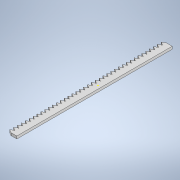
# Autodesk Inventor part: modelGateZoubkouváTyč
Saved by Autodesk Inventor 2020 (Build 240168000, 168)
## iProperties
Created: 2023-11-04
Part Number: modelGateZoubkouváTyč
Material: Generic
Document SubType Name: Sheet Metal
Designer: jirka
Density: 1 g/cm^3
Sheet Metal Rule: Default_mm
Appearance: Default
Author: jirka
Autodesk Inventor part; units mm, degrees
ref_plane "YZ Plane" through (0, 0, 0) normal (1, 0, 0) x (0, 1, 0)
ref_plane "XZ Plane" through (0, 0, 0) normal (0, 1, 0) x (-1, 0, 0)
ref_plane "XY Plane" through (0, 0, 0) normal (0, 0, 1) x (1, 0, 0)
sketch "Sketch1" plane through (0, 0, 0) normal (0, 1, 0) x (-1, 0, 0)
  line L0 (2.25, 55) -> (-2.25, 55)
  line L1 (-2.25, 55) -> (-2.25, -55)
  line L2 (-2.25, -55) -> (2.25, -55)
  line L3 (2.25, -55) -> (2.25, 55)
  point P0 (0, 0)
  dimension "d0" = 4.5
  dimension "d1" = 110
  dimension "d2" = 2.25
  dimension "d3" = 55
  constraints: 8 end point, 2 parallel, 1 horizontal, 1 perpendicular
  measures "d0" distance of L2.end L1.end
  measures "d1" distance of L1.end L0.end
  measures "d2" distance from line of L3 point (0, 0)
  measures "d3" distance from line of L0 point (0, 0)
extrude "Extrusion1" add sketch "Sketch1" along normal blind 2
sketch "Sketch2" plane through (0, 2, 0) normal (0, 1, 0) x (1, 0, 0)
  line L0 (-2.25, 55) -> (-2.25, -55) projected
  line L1 (-2.25, -55) -> (-3.2, -55)
  line L2 (-3.2, -55) -> (-3.2, -53)
  line L3 (-3.2, -53) -> (-2.25, -53)
  line L4 (-2.25, -53) -> (-2.25, -55)
  line L5 (-2.25, -55) -> (-3.2, -54)
  line L6 (-2.25, -53) -> (-3.2, -54)
  line L7 (-3.2, -54) -> (-2.25, -54)
  line L8 (-2.25, -54) -> (-2.513, -54)
  circle A0 centre (-2.513, -54) radius 0.5
  point P0 (0, 0)
  point P1 (-2.9043, -53.6887)
  point P2 (-2.9043, -54.3113)
  dimension "d6" = 0.263
  dimension "d7" = 1
  constraints: 16 end point, 2 midpoint, 2 parallel, 1 centre point, 1 coincident, 1 horizontal, 1 perpendicular, 1 point on line
  measures "d6" distance of L7.end L8.end
  measures "d7" diameter of A0
extrude "Extrusion2" add sketch "Sketch2" against normal blind 2 contours L0 A0 L6 | L0 L7 A0 | L0 A0 L7 | L0 L5 A0
pattern_linear "Rectangular Pattern1" count 55 spacing 2 along (0, 0, -1) of "Extrusion2"
sketch "Sketch3" plane through (0, 0, 0) normal (0, -1, 0) x (1, 0, 0)
  line L0 (2.25, -55) -> (-2.25, -55) projected
  line L1 (-2.25, 55) -> (-2.9043, 54.3113) projected
  line L2 (-2.25, -55) -> (-2.25, 55)
  line L3 (-2.25, -55) -> (-2.25, -52)
  line L4 (-2.25, -53.5) -> (-4.75, -53.5)
  line L5 (-2.25, -52) -> (-4.75, -53.5)
  line L6 (-4.75, -53.5) -> (-2.25, -55)
  point P0 (0, 0)
  point P1 (-3.5, -52.75)
  point P2 (-3.5, -54.25)
  dimension "d13" = 3
  constraints: 10 end point, 3 midpoint, 1 horizontal, 1 point on line, 1 vertical
  measures "d13" distance of L0.end L3.end
extrude "Extrusion3" add sketch "Sketch3" against normal up to surface (2 mm away)
sketch "Sketch4" plane through (0, 0, 0) normal (0, -1, 0) x (1, 0, 0)
  line L0 (2.25, -55) -> (-2.25, -55) projected
  line L1 (-2.9043, 54.3113) -> (-2.25, 55) projected
  line L2 (-2.25, -55) -> (-2.25, 55)
  line L3 (-2.8551, -52.3631) -> (-4.75, -53.5) projected
  line L4 (-3.0991, -52.5094) -> (-2.25, -52)
  line L5 (-3.0991, -52.5094) -> (-8.5995, 61.032)
  line L6 (-2.25, 55) -> (-8.5995, 61.032)
  point P0 (0, 0)
  point P1 (-3.5, -52.75)
  point P2 (-2.8551, -52.3631)
  constraints: 8 end point, 2 point on line, 1 collinear, 1 vertical
extrude "Extrusion4" cut sketch "Sketch4" against normal blind 10
pattern_linear "Rectangular Pattern2" count 40 spacing 3 along (0, 0, 1) of "Extrusion3"
sketch "Sketch5" plane through (-2.25, 0, 59) normal (1, 0, 0) x (0, 0, -1)
  line L0 (-6, 0) -> (-6, 2) projected
  line L1 (5.25, 2) -> (6, 2) projected
  line L2 (-6, 0) -> (5.25, 0)
  line L3 (5.25, 0) -> (5.25, 2)
  line L4 (5.25, 2) -> (-6, 2)
  line L5 (-6, 2) -> (-6, 0)
  point P0 (59, 0)
  constraints: 8 end point, 2 parallel, 1 horizontal, 1 perpendicular
extrude "Extrusion5" [suppressed]
sketch "Sketch6" plane through (0, 0, 0) normal (0, -1, 0) x (1, 0, 0)
  point P0 (0, 0)
sketch "Sketch7" plane through (2.25, 0, 55) normal (0, 0, 1) x (1, 0, 0)
  line L0 (-4.5, 0) -> (-4.5, 2) projected
  line L1 (0, 0) -> (0, 2) projected
  line L2 (-4.5, 0) -> (0, 0)
  line L3 (0, 0) -> (0, 2)
  line L4 (0, 2) -> (-4.5, 2)
  line L5 (-4.5, 2) -> (-4.5, 0)
  point P0 (-2.25, 0)
  point P1 (0, 0)
  constraints: 8 end point, 2 parallel, 1 horizontal, 1 perpendicular
extrude "Extrusion6" add sketch "Sketch7" along normal blind 10
sketch "Sketch8" plane through (0, 2, 0) normal (0, 1, 0) x (1, 0, 0)
  point P0 (0, 0)
equation "\"d2\" = 0.5 * d0"
equation "\"BendRadius\" = Thickness"
equation "\"BendReliefWidth\" = Thickness"
equation "\"BendReliefDepth\" = 0.5 * Thickness"
equation "\"CornerReliefSize\" = 4 * Thickness"
equation "\"MinimumRemnant\" = 2 * Thickness"
equation "\"TransitionRadius\" = BendRadius"
equation "\"JacobiRadiusSize\" = BendRadius"
equation "\"GapSize\" = Thickness"
equation "\"Thickness\" = 0.5"
body "Solid1"
